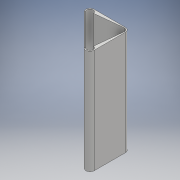
# Autodesk Inventor part: Cage30mm-2sides-L100mm
Saved by Autodesk Inventor 2017 (Build 210142000, 142)
## iProperties
Created: 2022-04-01
Part Number: Cage30mm-2sides-L100mm
Material: Generic
Document SubType Name: Modeling
Designer: Nikita
Density: 1 g/cm^3
Appearance: Default
Author: Nikita
Autodesk Inventor part; units mm, degrees
ref_plane "YZ Plane" through (0, 0, 0) normal (1, 0, 0) x (0, 1, 0)
ref_plane "XZ Plane" through (0, 0, 0) normal (0, 1, 0) x (-1, 0, 0)
ref_plane "XY Plane" through (0, 0, 0) normal (0, 0, 1) x (1, 0, 0)
sketch "Sketch2" plane through (0, 0, 0) normal (0, 0, 1) x (1, 0, 0)
  arc A0 (-11.9166, 15.3203) -> (-17.192, 12.808) centre (-15, 15) ccw
  arc A1 (18.0834, 14.6797) -> (14.6797, 18.0834) centre (15, 15) ccw
  arc A2 (12.808, -17.192) -> (15.3203, -11.9166) centre (15, -15) ccw
  arc A3 (12.1716, -17.8284) -> (15.4133, -11.0214) centre (15, -15) ccw
  line L0 (-15, 19) -> (15, 19)
  line L1 (19, 15) -> (19, -15)
  line L2 (-15, 15) -> (-17.8284, 12.1716)
  line L3 (-15, 15) -> (-11, 15) construction
  line L4 (-15, 15) -> (14.6797, 18.0834)
  line L5 (15, -15) -> (18.0834, 14.6797)
  line L6 (15, -15) -> (12.1716, -17.8284)
  arc A4 (-11.0214, 15.4133) -> (-17.8284, 12.1716) centre (-15, 15) ccw
  arc A5 (19, 15) -> (15, 19) centre (15, 15) ccw
  point P0 (0, 0)
  dimension "d18" = 6.2
  dimension "d19" = 6.2
  dimension "d22" = 8
  dimension "d24" = 135
  constraints: 14 end point, 14 point on circle, 6 centre point, 6 coincident, 6 point on line, 4 tangent, 1 equal length, 1 horizontal
  measures "d18" diameter of A1
  measures "d19" diameter of A2
  measures "d22" diameter of A3
  measures "d24" angle of L2 L3
extrude "Extrusion2" add sketch "Sketch2" along normal blind 100 contours A0 L2 A4 L4 | A4 L0 A5 L1 A3 L5 A1 L4 | A3 L6 A2 L5
body "Solid2"
